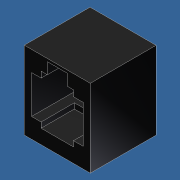
# Autodesk Inventor part: 2009_CTS_EatherNetPort
Saved by Autodesk Inventor 2012 (Build 160160000, 160)
## iProperties
Company: Team 801
Created: 2009-01-31
Part Number: 2009_CTS_EatherNetPort
Document SubType Name: Modeling
Designer: Jeffrey M
Density: 1 g/cm^3
Material: Default
Mass: 1.46941 g
Surface Area: 18.0832 cm^2
Volume: 1.46941 cm^3
Title: 2009_CTS_EatherNetPort
Author: Jeffrey M
Autodesk Inventor part; units mm, degrees
ref_plane "YZ Plane" through (0, 0, 0) normal (1, 0, 0) x (0, 1, 0)
ref_plane "XZ Plane" through (0, 0, 0) normal (0, 1, 0) x (-1, 0, 0)
ref_plane "XY Plane" through (0, 0, 0) normal (0, 0, 1) x (1, 0, 0)
sketch "Sketch1" plane through (0, 0, 0) normal (0, 0, 1) x (1, 0, 0)
  line L0 (-15.1032, 11.1381) -> (-28.4636, 11.1381)
  line L1 (-28.4636, 11.1381) -> (-28.4636, 26.8861)
  line L2 (-28.4636, 26.8861) -> (-15.1032, 26.8861)
  line L3 (-15.1032, 26.8861) -> (-15.1032, 11.1381)
  dimension "d0" = 13.3604
  dimension "d1" = 15.748
  constraints: 8 end point, 2 parallel, 1 horizontal, 1 perpendicular
  measures "d0" distance of L1.end L2.end
  measures "d1" distance of L2.end L0.start
extrude "Extrusion1" add sketch "Sketch1" along normal blind 13.3096
sketch "Sketch2" plane through (0, 0, 13.3096) normal (0, 0, 1) x (1, 0, 0)
  line L0 (-28.4636, 11.1381) -> (-28.4636, 26.8861) projected
  line L1 (-15.1032, 11.1381) -> (-28.4636, 11.1381) projected
  line L2 (-15.1032, 26.8861) -> (-15.1032, 11.1381) projected
  line L3 (-28.4636, 26.8861) -> (-15.1032, 26.8861) projected
  line L4 (-23.79, 26.3273) -> (-19.7768, 26.3273)
  line L5 (-19.7768, 26.3273) -> (-19.7768, 24.0413)
  line L6 (-19.7768, 24.0413) -> (-23.79, 24.0413)
  line L7 (-23.79, 24.0413) -> (-23.79, 26.3273)
  line L8 (-25.06, 24.0413) -> (-18.5068, 24.0413)
  line L9 (-18.5068, 24.0413) -> (-18.5068, 22.8221)
  line L10 (-18.5068, 22.8221) -> (-25.06, 22.8221)
  line L11 (-25.06, 22.8221) -> (-25.06, 24.0413)
  line L12 (-16.5764, 22.8221) -> (-26.9904, 22.8221)
  line L13 (-26.9904, 22.8221) -> (-26.9904, 15.1259)
  line L14 (-26.9904, 15.1259) -> (-16.5764, 15.1259)
  line L15 (-16.5764, 15.1259) -> (-16.5764, 22.8221)
  line L16 (-25.06, 15.1259) -> (-18.5068, 15.1259)
  line L17 (-18.5068, 15.1259) -> (-18.5068, 14.0337)
  line L18 (-18.5068, 14.0337) -> (-25.06, 14.0337)
  line L19 (-25.06, 14.0337) -> (-25.06, 15.1259)
  dimension "d4" = 0.5588
  dimension "d5" = 4.6736
  dimension "d6" = 4.6736
  dimension "d7" = 2.286
  dimension "d9" = 1.27
  dimension "d10" = 1.27
  dimension "d11" = 1.2192
  dimension "d13" = 6.5532
  dimension "d14" = 1.9304
  dimension "d15" = 1.9304
  dimension "d16" = 10.414
  dimension "d17" = 7.6962
  dimension "d18" = 1.9304
  dimension "d19" = 1.9304
  dimension "d20" = 1.0922
  dimension "d21" = 2.8956
  constraints: 32 end point, 8 parallel, 4 horizontal, 4 perpendicular, 1 point on line
  measures "d4" distance between parallel lines of L3 L4
  measures "d5" distance between parallel lines of L2 L5
  measures "d6" distance between parallel lines of L0 L7
  measures "d7" distance of L4.end L5.end
  measures "d9" distance of L6.end L8.start
  measures "d10" distance of L5.end L8.end
  measures "d11" distance of L10.end L8.start
  measures "d13" distance of L8.start L8.end
  measures "d14" distance of L10.end L12.end
  measures "d15" distance of L12.start L9.end
  measures "d16" distance of L12.start L12.end
  measures "d17" distance of L14.end L12.start
  measures "d18" distance of L13.end L16.start
  measures "d19" distance of L14.end L16.end
  measures "d20" distance of L16.end L17.end
  measures "d21" distance between parallel lines of L1 L18
extrude "Extrusion2" cut sketch "Sketch2" against normal blind 14.1478 contours L4 L5 L6 L7 | L6 L8 L9 L10 L11 | L10 L12 L15 L14 L13 | L14 L17 L18 L19
sketch "Sketch3" plane through (0, 0, 0) normal (0, 0, -1) x (-1, 0, 0)
  line L0 (15.1032, 11.1381) -> (28.4636, 11.1381) projected
  line L1 (28.4636, 11.1381) -> (28.4636, 26.8861) projected
  line L2 (28.4636, 26.8861) -> (15.1032, 26.8861) projected
  line L3 (15.1032, 26.8861) -> (15.1032, 11.1381) projected
extrude "Extrusion3" add sketch "Sketch3" against normal blind 0.127
sketch "Sketch4" plane through (0, 0, 0.127) normal (0, 0, 1) x (1, 0, 0)
  line L0 (-25.06, 14.0337) -> (-25.06, 15.1259) projected
  line L1 (-18.5068, 14.0337) -> (-25.06, 14.0337) projected
  line L2 (-18.5068, 15.1259) -> (-18.5068, 14.0337) projected
  line L3 (-22.8629, 14.0337) -> (-22.6089, 14.0337)
  line L4 (-22.6089, 14.0337) -> (-22.6089, 16.4931)
  line L5 (-22.6089, 16.4931) -> (-22.8629, 16.4931)
  line L6 (-22.8629, 16.4931) -> (-22.8629, 14.0337)
  line L7 (-22.2279, 14.0337) -> (-21.9739, 14.0337)
  line L8 (-21.9739, 14.0337) -> (-21.9739, 16.4931)
  line L9 (-21.9739, 16.4931) -> (-22.2279, 16.4931)
  line L10 (-22.2279, 16.4931) -> (-22.2279, 14.0337)
  line L11 (-21.5929, 14.0337) -> (-21.3389, 14.0337)
  line L12 (-21.3389, 14.0337) -> (-21.3389, 16.4931)
  line L13 (-21.3389, 16.4931) -> (-21.5929, 16.4931)
  line L14 (-21.5929, 16.4931) -> (-21.5929, 14.0337)
  line L15 (-20.9579, 14.0337) -> (-20.7039, 14.0337)
  line L16 (-20.7039, 14.0337) -> (-20.7039, 16.4931)
  line L17 (-20.7039, 16.4931) -> (-20.9579, 16.4931)
  line L18 (-20.9579, 16.4931) -> (-20.9579, 14.0337)
  dimension "d26" = 0.254
  dimension "d27" = 0.254
  dimension "d28" = 0.254
  dimension "d29" = 0.254
  dimension "d30" = 0.381
  dimension "d31" = 0.381
  dimension "d32" = 0.381
  dimension "d33" = 2.1971
  dimension "d34" = 2.1971
  constraints: 32 end point, 8 parallel, 4 horizontal, 4 perpendicular, 4 point on line
  measures "d26" distance of L16.end L17.end
  measures "d27" distance of L12.end L13.end
  measures "d28" distance of L8.end L9.end
  measures "d29" distance of L4.end L5.end
  measures "d30" distance between parallel lines of L18 L12
  measures "d31" distance between parallel lines of L8 L14
  measures "d32" distance between parallel lines of L10 L4
  measures "d33" distance between parallel lines of L2 L16
  measures "d34" distance between parallel lines of L0 L6
extrude "Extrusion4" add sketch "Sketch4" along normal blind 6.4516
sketch "Sketch5" plane through (-22.8629, 14.0337, 0.127) normal (-1, 0, 0) x (0, 0, 1)
  line L0 (6.4516, 0) -> (6.4516, 2.4594) projected
  line L1 (0, 2.4594) -> (6.4516, 2.4594) projected
  line L2 (6.4516, 0) -> (0.1115, 2.4594)
  constraints: 2 end point, 1 point on line
extrude "Extrusion5" cut sketch "Sketch5" against normal blind 3.81
fillet "Fillet1" radius 0.127 8 edges at (-22.8629, 15.2634, 3.4085) (-22.6089, 15.2634, 3.4085) (-21.9739, 15.2634, 3.4085) (-22.2279, 15.2634, 3.4085) (-21.5929, 15.2634, 3.4085) (-21.3389, 15.2634, 3.4085) (-20.9579, 15.2634, 3.4085) (-20.7039, 15.2634, 3.4085)
sketch "Sketch6" plane through (0, 0, 0.127) normal (0, 0, 1) x (1, 0, 0)
  line L0 (-22.6089, 16.4001) -> (-22.6089, 14.0337) projected
  line L1 (-21.9739, 16.4001) -> (-21.9739, 14.0337) projected
  line L2 (-21.3389, 16.4001) -> (-21.3389, 14.0337) projected
  line L3 (-20.7039, 16.4001) -> (-20.7039, 14.0337) projected
  line L4 (-18.5068, 14.0337) -> (-20.7039, 14.0337) projected
  line L5 (-22.8629, 14.0337) -> (-25.06, 14.0337) projected
  line L6 (-22.8629, 14.0337) -> (-22.8629, 16.4001) projected
  line L7 (-25.0727, 14.0337) -> (-22.8629, 14.0337)
  line L8 (-22.8629, 14.0337) -> (-22.8629, 15.1259)
  line L9 (-22.8629, 15.1259) -> (-25.0727, 15.1259)
  line L10 (-25.0727, 15.1259) -> (-25.0727, 14.0337)
  line L11 (-22.6089, 15.1259) -> (-22.2279, 15.1259)
  line L12 (-22.2279, 15.1259) -> (-22.2279, 14.0337)
  line L13 (-22.2279, 14.0337) -> (-22.6089, 14.0337)
  line L14 (-22.6089, 14.0337) -> (-22.6089, 15.1259)
  line L15 (-21.9739, 15.1259) -> (-21.5929, 15.1259)
  line L16 (-21.5929, 15.1259) -> (-21.5929, 14.0337)
  line L17 (-21.5929, 14.0337) -> (-21.9739, 14.0337)
  line L18 (-21.9739, 14.0337) -> (-21.9739, 15.1259)
  line L19 (-21.3389, 15.1259) -> (-20.9579, 15.1259)
  line L20 (-20.9579, 15.1259) -> (-20.9579, 14.0337)
  line L21 (-20.9579, 14.0337) -> (-21.3389, 14.0337)
  line L22 (-21.3389, 14.0337) -> (-21.3389, 15.1259)
  line L23 (-20.7039, 15.1259) -> (-18.4941, 15.1259)
  line L24 (-18.4941, 15.1259) -> (-18.4941, 14.0337)
  line L25 (-18.4941, 14.0337) -> (-20.7039, 14.0337)
  line L26 (-20.7039, 14.0337) -> (-20.7039, 15.1259)
  line L27 (-22.8629, 14.0337) -> (-25.0727, 14.0337)
  line L28 (-25.0727, 14.0337) -> (-25.0727, 15.1259)
  line L29 (-25.0727, 15.1259) -> (-22.8629, 15.1259)
  line L30 (-22.8629, 15.1259) -> (-22.8629, 14.0337)
  line L31 (-20.7039, 15.1259) -> (-18.4941, 15.1259)
  line L32 (-18.4941, 15.1259) -> (-18.4941, 14.0337)
  line L33 (-18.4941, 14.0337) -> (-20.7039, 14.0337)
  line L34 (-20.7039, 14.0337) -> (-20.7039, 15.1259)
  point P0 (-25.06, 15.1259)
  dimension "d40" = 1.0922
  dimension "d41" = 1.0922
  dimension "d42" = 0
  dimension "d43" = 0
  dimension "d44" = 0
  dimension "d45" = 0
  dimension "d46" = 2.2098
  dimension "d47" = 2.2098
  constraints: 56 end point, 14 parallel, 7 horizontal, 7 perpendicular, 7 point on line
  measures "d40" distance between parallel lines of L13 L11
  measures "d41" distance of L5.end point (-25.06, 15.126)
  measures "d42" distance from line of L11.start L9
  measures "d43" distance between parallel lines of L11 L15
  measures "d44" distance between parallel lines of L15 L23
  measures "d45" distance between parallel lines of L23 L19
  measures "d46" distance of L8.end L9.end
  measures "d47" distance of L23.start L23.end
extrude "Extrusion6" add sketch "Sketch6" along normal blind 6.4516
sketch "Sketch7" plane through (0, 0, 0.127) normal (0, 0, 1) x (1, 0, 0)
  line L0 (-22.8629, 15.1259) -> (-22.6089, 15.1259)
  line L1 (-22.6089, 15.1259) -> (-22.6089, 22.5284)
  line L2 (-22.6089, 22.5284) -> (-22.8629, 22.5284)
  line L3 (-22.8629, 22.5284) -> (-22.8629, 15.1259)
  line L4 (-22.2279, 15.1259) -> (-21.9739, 15.1259)
  line L5 (-21.9739, 15.1259) -> (-21.9739, 22.5284)
  line L6 (-21.9739, 22.5284) -> (-22.2279, 22.5284)
  line L7 (-22.2279, 22.5284) -> (-22.2279, 15.1259)
  line L8 (-21.5929, 15.1259) -> (-21.3389, 15.1259)
  line L9 (-21.3389, 15.1259) -> (-21.3389, 22.5284)
  line L10 (-21.3389, 22.5284) -> (-21.5929, 22.5284)
  line L11 (-21.5929, 22.5284) -> (-21.5929, 15.1259)
  line L12 (-20.9579, 15.1259) -> (-20.7039, 15.1259)
  line L13 (-20.7039, 15.1259) -> (-20.7039, 22.5284)
  line L14 (-20.7039, 22.5284) -> (-20.9579, 22.5284)
  line L15 (-20.9579, 22.5284) -> (-20.9579, 15.1259)
  line L16 (-22.9407, 16.4931) -> (-20.3193, 16.4931)
  line L17 (-20.7381, 16.4931) -> (-20.9579, 16.4931)
  line L18 (-20.9579, 16.4931) -> (-20.9579, 22.5284)
  line L19 (-20.9579, 22.5284) -> (-20.7381, 22.5284)
  line L20 (-21.5929, 22.5284) -> (-21.3731, 22.5284)
  line L21 (-21.3731, 16.4931) -> (-21.5929, 16.4931)
  line L22 (-21.5929, 16.4931) -> (-21.5929, 22.5284)
  line L23 (-20.7039, 16.4931) -> (-20.9579, 16.4931)
  line L24 (-20.9579, 16.4931) -> (-20.9579, 22.5284)
  line L25 (-20.9579, 22.5284) -> (-20.7039, 22.5284)
  line L26 (-20.7039, 22.5284) -> (-20.7039, 16.4931)
  line L27 (-21.5929, 22.5284) -> (-21.3389, 22.5284)
  line L28 (-21.3389, 22.5284) -> (-21.3389, 16.4931)
  line L29 (-21.3389, 16.4931) -> (-21.5929, 16.4931)
  line L30 (-21.5929, 16.4931) -> (-21.5929, 22.5284)
  line L31 (-21.9739, 16.4931) -> (-22.2279, 16.4931)
  line L32 (-22.2279, 16.4931) -> (-22.2279, 22.5284)
  line L33 (-22.2279, 22.5284) -> (-21.9739, 22.5284)
  line L34 (-21.9739, 22.5284) -> (-21.9739, 16.4931)
  line L35 (-22.8629, 22.5284) -> (-22.6089, 22.5284)
  line L36 (-22.6089, 22.5284) -> (-22.6089, 16.4931)
  line L37 (-22.6089, 16.4931) -> (-22.8629, 16.4931)
  line L38 (-22.8629, 16.4931) -> (-22.8629, 22.5284)
  constraints: 78 end point, 18 parallel, 10 horizontal, 10 perpendicular, 8 point on line
extrude "Extrusion7" cut sketch "Sketch7" against normal blind 127 contours L15 L14 L13 L16 | L11 L10 L9 L16 | L7 L6 L5 L16 | L3 L2 L1 L16
equation "\"d6\" = d5"
equation "\"d10\" = d9"
equation "\"d15\" = d14"
equation "\"d27\" = d26"
equation "\"d28\" = d27"
equation "\"d29\" = d28"
equation "\"d31\" = d30"
equation "\"d32\" = d31"
equation "\"d40\" = d41"
equation "\"d47\" = d46"
body "Solid1"
